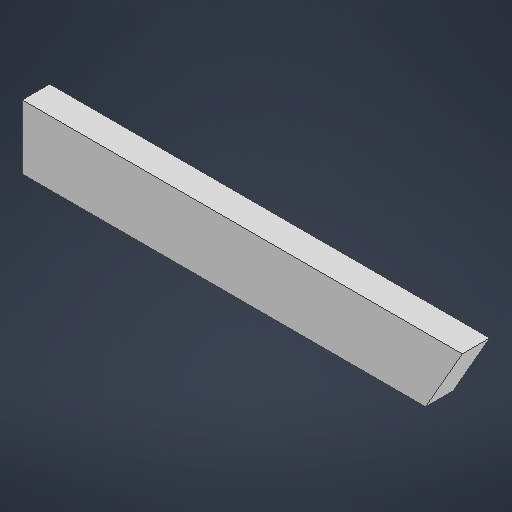
# Autodesk Inventor part: S_2x4x24
Saved by Autodesk Inventor 2026 (Build 300175000, 175)
## iProperties
Created: 2025-09-02
Part Number: S_2x4x24
Material: Generic
Document SubType Name: Modeling
Designer: trott
Density: 1 g/cm^3
Appearance: Default
Author: trott
Autodesk Inventor part; units mm, degrees
ref_plane "YZ Plane" through (0, 0, 0) normal (1, 0, 0) x (0, 1, 0)
ref_plane "XZ Plane" through (0, 0, 0) normal (0, 1, 0) x (-1, 0, 0)
ref_plane "XY Plane" through (0, 0, 0) normal (0, 0, 1) x (1, 0, 0)
sketch "Sketch1" plane through (0, 0, 0) normal (0, 0, 1) x (1, 0, 0)
  line L0 (-609.6, -1371.6) -> (609.6, -1371.6)
  line L1 (609.6, -1371.6) -> (609.6, 1371.6)
  line L2 (609.6, 1371.6) -> (-609.6, 1371.6)
  line L3 (-609.6, 1371.6) -> (-609.6, -1371.6)
  line L4 (-609.6, -1371.6) -> (609.6, 1371.6) construction
  line L5 (609.6, -1371.6) -> (-609.6, 1371.6) construction
  line L6 (0, -304.8) -> (609.6, -304.8)
  line L7 (0, -1371.6) -> (609.6, -304.8)
  line L8 (0, 1371.6) -> (609.6, -304.8)
  line L9 (0, -304.8) -> (0, -393.7)
  line L10 (0, -393.7) -> (558.8, -393.7)
  line L11 (609.6, -304.8) -> (520.7, -304.8)
  point P0 (0, 0)
  dimension "d0" = 1219.2
  dimension "d1" = 2743.2
  dimension "d2" = 304.8
  dimension "d4" = 88.9
  constraints: 24 end point, 4 midpoint, 3 perpendicular, 3 point on line, 2 parallel, 1 horizontal, 1 vertical
  measures "d0" distance of L1.end L2.end
  measures "d1" distance of L0.end L1.end
  measures "d2" distance of point (0, 0) L6.start
  measures "d4" distance of L6.start L9.end
extrude "Extrusion1" add sketch "Sketch1" along normal blind 38.1 contours L10 L9 L6 L7
body "Solid1"
